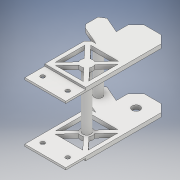
# Autodesk Inventor part: Forearm1 v2
Saved by Autodesk Inventor 2018 (Build 220112000, 112)
## iProperties
Created: 2018-04-13
Part Number: Forearm1 v2
Material: Plastique ABS
Document SubType Name: Modeling
Designer: Thomas
Density: 1.06 g/cm^3
Appearance: Lisse - Blanc
Author: Thomas
Autodesk Inventor part; units mm, degrees
ref_plane "YZ Plane" through (0, 0, 0) normal (1, 0, 0) x (0, 1, 0)
ref_plane "XZ Plane" through (0, 0, 0) normal (0, 1, 0) x (-1, 0, 0)
ref_plane "XY Plane" through (0, 0, 0) normal (0, 0, 1) x (1, 0, 0)
sketch "Esquisse2" plane through (0, 0, 0) normal (0, 0, 1) x (1, 0, 0)
  line L0 (0, 0) -> (41.5, 0)
  line L1 (41.5, 0) -> (41.5, -41.5)
  line L2 (0, 0) -> (41.5, -41.5) construction
  circle A0 centre (20.7915, -20.7085) radius 5
  line L3 (0, -25) -> (-20.4662, -16.0249)
  line L4 (-27.4743, -20.6039) -> (-27.4743, -35.9516)
  line L5 (-27.4743, -35.9516) -> (-23.1441, -40.4516)
  line L6 (0, 0) -> (0, -25)
  line L7 (-23.1441, -40.4516) -> (0, -50.6933)
  line L8 (-20.4662, -16.0249) -> (-27.4743, -20.6039)
  line L9 (41.5, -41.5) -> (41.5, -50.6933)
  line L10 (0, -50.6933) -> (-5, -50.6933)
  line L11 (-10, -55.6933) -> (-10, -130)
  line L12 (-10, -130) -> (41.5, -130)
  line L13 (41.5, -130) -> (41.5, -50.6933)
  line L14 (-5, -50.6933) -> (-10, -55.6933)
  point P0 (-10, -50.6933)
  dimension "d0" = 41.5
  dimension "d1" = 41.5
  dimension "d2" = 10
  dimension "d32" = 25
  dimension "d45" = 10
  dimension "d46" = 5
  dimension "d47" = 5
  dimension "d48" = 130
  constraints: 30 end point, 4 vertical, 3 perpendicular, 2 horizontal, 2 point on line, 1 centre point
  measures "d0" distance of L0.start L0.end
  measures "d1" distance of L0.end L1.end
  measures "d2" diameter of A0
  measures "d32" distance of L0.start L3.start
  measures "d45" distance of L7.end point (-10, -50.693)
  measures "d46" distance of L10.end point (-10, -50.693)
  measures "d47" distance of L11.start point (-10, -50.693)
  measures "d48" distance between parallel lines of L0 L12
extrude "Extrusion3" add sketch "Esquisse2" along normal blind 5
sketch "Esquisse4" plane through (0, 0, 5) normal (0, 0, 1) x (1, 0, 0)
  circle A0 centre (-17.0573, -30.35) radius 5
  line L0 (0, -25) -> (-20.4662, -16.0249) projected
  point P0 (0, 0)
  dimension "d53" = 10
  dimension "d54" = 11.75
  constraints: 1 centre point
  measures "d53" diameter of A0
  measures "d54" distance from line of L0 A0.centre
extrude "Extrusion4" add sketch "Esquisse4" along normal blind 70
sketch "Esquisse5" plane through (-17.0573, -30.35, 75) normal (0, 0, 1) x (1, 0, 0)
  line L0 (17.0722, 30.4073) -> (58.5722, 30.4073)
  line L1 (58.5722, 30.4073) -> (58.5722, -11.0927)
  line L2 (17.0722, 5.4073) -> (-3.394, 14.3825)
  line L3 (-10.4021, 9.8034) -> (-10.4021, -5.5443)
  line L4 (-10.4021, -5.5443) -> (-6.072, -10.0443)
  line L5 (17.0722, 30.4073) -> (17.0722, 5.4073)
  line L6 (-6.072, -10.0443) -> (17.0722, -20.2859)
  line L7 (-3.394, 14.3825) -> (-10.4021, 9.8034)
  line L8 (58.5722, -11.0927) -> (58.5722, -20.2859)
  line L9 (17.0722, -20.2859) -> (12.0722, -20.2859)
  line L10 (7.0722, -25.2859) -> (7.0722, -99.5927)
  line L11 (7.0722, -99.5927) -> (58.5722, -99.5927)
  line L12 (58.5722, -99.5927) -> (58.5722, -20.2859)
  line L13 (12.0722, -20.2859) -> (7.0722, -25.2859)
  point P0 (17.0573, 30.35)
  point P1 (7.0722, -20.2859)
  dimension "d57" = 41.5
  dimension "d58" = 41.5
  dimension "d60" = 25
  dimension "d61" = 10
  dimension "d62" = 5
  dimension "d63" = 5
  dimension "d64" = 130
  constraints: 28 end point, 4 vertical, 3 perpendicular, 2 horizontal, 2 point on line
  measures "d57" distance of L0.start L1.start
  measures "d58" distance of L1.start L1.end
  measures "d60" distance of L0.start L2.start
  measures "d61" distance of L6.end point (7.072, -20.286)
  measures "d62" distance of L9.end point (7.072, -20.286)
  measures "d63" distance of L13.end point (7.072, -20.286)
  measures "d64" distance between parallel lines of L0 L11
chamfer "Chanfrein7" distance 10 angle 45 1 edges at (0, 0, 2.5)
chamfer "Chanfrein8" distance 10 angle 45 1 edges at (41.5, 0, 2.5)
extrude "Extrusion6" add sketch "Esquisse5" along normal blind 5
chamfer "Chanfrein9" distance 10 angle 45 1 edges at (41.5149, 0.0573, 77.5)
chamfer "Chanfrein10" distance 10 angle 45 1 edges at (0.0149, 0.0573, 77.5)
sketch "Esquisse6" plane through (0, 0, 0) normal (0, 0, -1) x (-1, 0, 0)
  line L0 (-41.5, -130) -> (9.9851, -130)
  line L1 (10, -105) -> (-41.5, -105)
  line L2 (-41.5, -105) -> (-41.5, -130)
  line L3 (9.7923, -105) -> (10, -105)
  line L4 (10, -130) -> (-41.5, -130) projected
  line L5 (9.8887, -130) -> (10, -130)
  line L6 (10, -130) -> (10, -55.6933) projected
  line L7 (10, -105) -> (10, -130)
  point P0 (0, 0)
  dimension "d87" = 25
  constraints: 12 end point, 2 collinear, 2 horizontal, 2 point on line, 1 parallel
  measures "d87" distance of L1.end L0.start
extrude "Extrusion7" cut sketch "Esquisse6" against normal blind 2.5
sketch "Esquisse7" plane through (0, 0, 2.5) normal (0, 0, -1) x (-1, 0, 0)
  circle A0 centre (-31.5, -117.5) radius 2.6
  line L0 (-41.5, -130) -> (-41.5, -105) projected
  line L1 (-41.5, -105) -> (10, -105) projected
  circle A1 centre (-0.0149, -117.5) radius 2.6
  line L2 (9.9851, -105) -> (9.9851, -130) projected
  point P0 (0, 0)
  dimension "d96" = 5.2
  dimension "d97" = 10
  dimension "d98" = 12.5
  dimension "d99" = 5.2
  dimension "d100" = 10
  constraints: 2 centre point
  measures "d96" diameter of A0
  measures "d97" distance from line of L0 A0.centre
  measures "d98" distance from line of L1 A0.centre
  measures "d99" diameter of A1
  measures "d100" distance from line of L2 A1.centre
extrude "Extrusion8" cut sketch "Esquisse7" against normal blind 2.5
sketch "Esquisse8" plane through (-17.0573, -30.35, 80) normal (0, 0, 1) x (1, 0, 0)
  line L0 (58.5573, -99.65) -> (58.5573, 20.35) projected
  line L1 (58.5573, -99.5927) -> (58.5573, -99.65)
  line L2 (7.0722, -99.65) -> (7.0722, -99.5927)
  line L3 (58.5722, -99.5927) -> (7.0722, -99.5927) projected
  line L4 (58.5722, -99.5927) -> (7.0722, -99.5927)
  line L5 (7.0722, -99.5927) -> (7.0722, -74.5927)
  line L6 (7.0722, -74.5927) -> (58.5722, -74.5927)
  line L7 (58.5722, -74.5927) -> (58.5722, -99.5927)
  point P0 (17.0573, 30.35)
  dimension "d103" = 25
  constraints: 12 end point, 3 parallel, 1 horizontal, 1 perpendicular
  measures "d103" distance of L4.end L5.end
extrude "Extrusion10" cut sketch "Esquisse8" against normal blind 2.5
sketch "Esquisse9" plane through (-17.0573, -30.35, 77.5) normal (0, 0, 1) x (1, 0, 0)
  circle A0 centre (17.0722, -87.15) radius 2.6 projected
  circle A1 centre (17.0722, -87.15) radius 2.6
  circle A2 centre (48.5573, -87.15) radius 2.6 projected
  circle A3 centre (48.5573, -87.15) radius 2.6
  point P0 (17.0573, 30.35)
  constraints: 2 centre point, 2 coincident
extrude "Extrusion11" cut sketch "Esquisse9" against normal blind 2.5
sketch "Esquisse10" plane through (0, 0, 0) normal (0, 0, -1) x (-1, 0, 0)
  line L0 (0, -50.6933) -> (9.9851, -50.6933) construction
  line L1 (9.9851, -50.6933) -> (9.9851, -105) construction
  line L2 (0, -50.6933) -> (-41.5, -50.6933) construction
  line L3 (-41.5, -10) -> (-41.5, -105) construction
  line L4 (-41.5, -105) -> (-41.5, -50.6933) construction
  line L5 (-31.0711, -55.6933) -> (4.9851, -55.6933)
  line L6 (4.9851, -55.6933) -> (4.9851, -100)
  line L7 (-31.0711, -55.6933) -> (-36.5, -55.6933)
  line L8 (-36.5, -55.6933) -> (-36.5, -59.2233) construction
  line L9 (-36.5, -55.6933) -> (-33.2298, -55.6933) construction
  line L10 (-41.5, -105) -> (9.9851, -105) construction
  line L11 (-36.5, -55.6933) -> (-36.5, -100)
  line L12 (-36.5, -100) -> (4.9851, -100)
  line L13 (-36.5, -55.6933) -> (4.9851, -100) construction
  line L14 (4.9851, -55.6933) -> (-36.5, -100) construction
  circle A0 centre (-15.7574, -77.8466) radius 7.5
  line L15 (-36.5, -100) -> (-36.5, -96.47) construction
  line L16 (-36.5, -100) -> (-32.97, -100) construction
  line L17 (-32.97, -100) -> (-18.6905, -84.7493)
  line L18 (-9.0624, -74.4663) -> (4.9851, -59.4633)
  line L19 (-12.5184, -71.0821) -> (1.8904, -55.6933)
  line L20 (-12.665, -84.6794) -> (1.6799, -100)
  line L21 (-8.98, -81.0585) -> (4.9851, -95.9735)
  line L22 (-36.5, -59.2233) -> (-36.5, -96.6948)
  line L23 (-32.7299, -55.6933) -> (1.8904, -55.6933)
  line L24 (4.9851, -59.4633) -> (4.9851, -95.9735)
  line L25 (1.6799, -100) -> (-32.97, -100)
  line L26 (-32.7299, -55.6933) -> (-18.5171, -70.8728)
  line L27 (-36.5, -59.4633) -> (-22.4232, -74.409)
  line L28 (-36.5, -96.6948) -> (-22.2945, -81.5231)
  point P0 (0, 0)
  point P1 (9.9851, -104.9427)
  point P2 (-41.5149, -104.9427)
  dimension "d57" = 41.5
  dimension "d58" = 41.5
  dimension "d60" = 25
  dimension "d61" = 10
  dimension "d62" = 5
  dimension "d63" = 5
  dimension "d64" = 130
  dimension "d118" = 15
  dimension "d110" = 5
  dimension "d111" = 5
  dimension "d116" = 5
  dimension "d117" = 5
  constraints: 56 end point, 13 point on line, 7 horizontal, 4 perpendicular, 1 collinear, 1 midpoint, 1 parallel, 1 vertical, 10 other
  measures "d110" distance between parallel lines of L2 L5
  measures "d111" distance from line of L1 L5.end
  measures "d116" distance between parallel lines of L11 L3
  measures "d117" distance from line of L10 L6.end
extrude "Extrusion12" cut sketch "Esquisse10" against normal blind 5 contours L5 L19 A0 L26 L7 | L6 L21 A0 L18 | A0 L28 L11 L27 | A0 L20 L12 L17
sketch "Esquisse11" plane through (-17.0573, -30.35, 80) normal (0, 0, 1) x (1, 0, 0)
  line L0 (48.5721, -20.2859) -> (58.5722, -20.2859) construction
  line L1 (58.5722, -20.2859) -> (58.5722, -74.5927) construction
  line L2 (48.5721, -20.2859) -> (7.0573, -20.2859) construction
  line L3 (17.501, -25.2859) -> (53.5722, -25.2859)
  line L4 (53.5722, -25.2859) -> (53.5722, -69.5927)
  line L5 (17.501, -25.2859) -> (12.0573, -25.2859)
  line L6 (12.0573, -25.2859) -> (12.0573, -28.8108) construction
  line L7 (12.0573, -25.2859) -> (15.3423, -25.2859) construction
  line L8 (7.0573, -74.5927) -> (58.5722, -74.5927) construction
  line L9 (12.0573, -25.2859) -> (12.0573, -69.5927)
  line L10 (12.0573, -69.5927) -> (53.5722, -69.5927)
  line L11 (12.0573, -25.2859) -> (53.5722, -69.5927) construction
  line L12 (53.5722, -25.2859) -> (12.0573, -69.5927) construction
  circle A0 centre (32.8147, -47.4393) radius 7.5
  line L13 (12.0573, -69.5927) -> (12.0573, -66.0575) construction
  line L14 (12.0573, -69.5927) -> (15.6035, -69.5927) construction
  line L15 (15.6035, -69.5927) -> (29.8797, -54.3412)
  line L16 (39.5079, -44.0553) -> (53.5722, -29.0303)
  line L17 (36.0535, -40.6747) -> (50.4623, -25.2859)
  line L18 (35.9101, -54.2708) -> (50.2563, -69.5927)
  line L19 (39.5942, -50.647) -> (53.5722, -65.5758)
  line L20 (12.0573, -28.8108) -> (12.0573, -66.2913)
  line L21 (15.8474, -25.2859) -> (50.4623, -25.2859)
  line L22 (53.5722, -29.0303) -> (53.5722, -65.5758)
  line L23 (50.2563, -69.5927) -> (15.6035, -69.5927)
  line L24 (15.8474, -25.2859) -> (30.0589, -40.464)
  line L25 (12.0573, -29.0404) -> (26.1489, -44.0018)
  line L26 (12.0573, -66.2913) -> (26.2734, -51.1082)
  line L27 (58.5722, -74.5927) -> (58.5722, 20.4073) projected
  line L28 (7.0722, -74.5927) -> (58.5722, -74.5927) projected
  line L29 (17.0722, -20.2859) -> (12.0722, -20.2859) projected
  line L30 (7.0722, -25.2859) -> (7.0722, -74.5927) projected
  line L31 (12.0573, -29.0404) -> (12.0573, -66.2913)
  point P0 (17.0573, 30.35)
  point P1 (0, 0)
  point P2 (58.5572, -74.5302)
  point P3 (7.0572, -74.5302)
  dimension "d127" = 15
  dimension "d123" = 5
  dimension "d124" = 5
  dimension "d126" = 5
  dimension "d128" = 0
  dimension "d129" = 0
  dimension "d130" = 0
  constraints: 56 end point, 12 point on line, 7 horizontal, 3 perpendicular, 2 collinear, 1 midpoint, 1 vertical, 10 other
  measures "d123" distance between parallel lines of L2 L3
  measures "d124" distance from line of L1 L3.end
  measures "d126" distance from line of L8 L4.end
  measures "d128" distance between parallel lines of L27 L1
  measures "d129" distance between parallel lines of L28 L8
  measures "d130" distance between parallel lines of L29 L2
extrude "Extrusion13" cut sketch "Esquisse11" against normal blind 5 contours L3 L17 A0 L24 L5 | L4 L19 A0 L16 | A0 L26 L9 L25 | A0 L18 L10 L15
sketch "Esquisse14" plane through (-17.0573, -30.35, 75) normal (0, 0, -1) x (-1, 0, 0)
  arc A0 (-39.5079, -44.0553) -> (-39.5942, -50.647) centre (-32.8147, -47.4393) ccw projected
  circle A1 centre (-32.8147, -47.4393) radius 5
  point P0 (-17.0573, 30.35)
  dimension "d136" = 10
  constraints: 1 centre point, 1 coincident
  measures "d136" diameter of A1
extrude "Extrusion14" add sketch "Esquisse14" along normal blind 70
equation "\"d47\" = d46"
equation "\"d63\" = d62"
